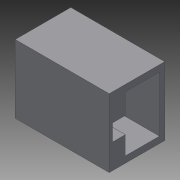
# Autodesk Inventor part: netwerk
Saved by Autodesk Inventor 2015 (Build 190159000, 159)
## iProperties
Created: 2015-12-03
Part Number: netwerk
Material: Generic
Document SubType Name: Modeling
Designer: david
Density: 1 g/cm^3
Appearance: Default
Author: david
Autodesk Inventor part; units mm, degrees
ref_plane "YZ Plane" through (0, 0, 0) normal (1, 0, 0) x (0, 1, 0)
ref_plane "XZ Plane" through (0, 0, 0) normal (0, 1, 0) x (-1, 0, 0)
ref_plane "XY Plane" through (0, 0, 0) normal (0, 0, 1) x (1, 0, 0)
sketch "Sketch1" plane through (0, 0, 0) normal (0, 1, 0) x (-1, 0, 0)
  line L0 (-11, 8) -> (11, 8)
  line L1 (11, 8) -> (11, -8)
  line L2 (11, -8) -> (-11, -8)
  line L3 (-11, -8) -> (-11, 8)
  line L4 (-11, 8) -> (11, -8) construction
  line L5 (11, 8) -> (-11, -8) construction
  point P0 (0, 0)
  dimension "d0" = 22
  dimension "d1" = 16
  constraints: 12 end point, 2 midpoint, 2 parallel, 1 horizontal, 1 perpendicular
  measures "d0" distance of L1.end L2.end
  measures "d1" distance of L0.end L1.end
extrude "Extrusion1" add sketch "Sketch1" along normal blind 13
sketch "Sketch2" plane through (11, 0, 8) normal (1, 0, 0) x (0, 0, -1)
  line L0 (1.5, 11.7761) -> (14.5, 11.7761)
  line L1 (14.5, 11.7761) -> (14.5, 3.7761)
  line L2 (14.5, 3.7761) -> (1.5, 3.7761)
  line L3 (1.5, 3.7761) -> (1.5, 11.7761)
  line L4 (0, 0) -> (0, 13) projected
  line L5 (6.3059, 3.7761) -> (10.1899, 3.7761)
  line L6 (10.1899, 3.7761) -> (10.1899, 0.7851)
  line L7 (10.1899, 0.7851) -> (6.3059, 0.7851)
  line L8 (6.3059, 0.7851) -> (6.3059, 3.7761)
  point P0 (8, 0)
  dimension "d4" = 13
  dimension "d5" = 8
  dimension "d6" = 1.5
  constraints: 16 end point, 4 parallel, 2 horizontal, 2 perpendicular, 1 point on line
  measures "d4" distance of L1.end L2.end
  measures "d5" distance of L0.end L1.end
  measures "d6" distance between parallel lines of L3 L4
extrude "Extrusion2" cut sketch "Sketch2" against normal blind 16
body "Solid1"
